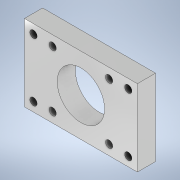
# Autodesk Inventor part: Techo Espaciador Sub. Inferior
Saved by Autodesk Inventor 2020 (Build 240168000, 168)
## iProperties
Created: 2020-05-16
Part Number: Techo Espaciador Sub. Inferior
Material: Aluminum 6061
Document SubType Name: Modeling
Designer: Dante
Density: 2.7 g/cm^3
Appearance: Aluminum - Dark
Mass: 53.2586 g
Surface Area: 78.472 cm^2
Volume: 19.7254 cm^3
Author: Dante
Autodesk Inventor part; units mm, degrees
ref_plane "YZ Plane" through (0, 0, 0) normal (1, 0, 0) x (0, 1, 0)
ref_plane "XZ Plane" through (0, 0, 0) normal (0, 1, 0) x (-1, 0, 0)
ref_plane "XY Plane" through (0, 0, 0) normal (0, 0, 1) x (1, 0, 0)
sketch "Sketch1" plane through (0, 0, 0) normal (0, 0, 1) x (1, 0, 0)
  line L0 (0, 0) -> (0, -42)
  line L1 (0, -42) -> (62, -42)
  line L2 (62, -42) -> (62, 0)
  line L3 (62, 0) -> (0, 0)
  line L4 (11, -42) -> (53, -42)
  line L5 (53, 0) -> (11, 0)
  line L6 (10, -5.9896) -> (10, -30.0104)
  line L7 (31, 0) -> (31, -13)
  circle A0 centre (5, -5) radius 2
  line L8 (0, -21) -> (-21.0238, -21)
  circle A1 centre (31, -21) radius 13
  circle A2 centre (15.5, -5.5) radius 2
  circle A3 centre (15.5, -36.5) radius 2
  circle A4 centre (5, -37) radius 2
  line L9 (52, -5.9896) -> (52, -30.0104)
  circle A5 centre (57, -5) radius 2
  circle A6 centre (46.5, -5.5) radius 2
  circle A7 centre (46.5, -36.5) radius 2
  circle A8 centre (57, -37) radius 2
  dimension "d0" = 42
  dimension "d1" = 62
  dimension "d42" = 10
  dimension "d43" = 4
  dimension "d44" = 5
  dimension "d45" = 5
  dimension "d46" = 26
  dimension "d47" = 4
  dimension "d50" = 4
  dimension "d51" = 5.5
  dimension "d52" = 5.5
  dimension "d53" = 5.5
  dimension "d54" = 31
  constraints: 20 end point, 9 centre point, 7 symmetric about line, 4 perpendicular, 2 vertical, 1 horizontal, 1 midpoint, 1 parallel, 1 point on line, 5 other
  measures "d0" distance of L0.start L0.end
  measures "d1" distance of L0.end L1.end
  measures "d42" distance between parallel lines of L0 L6
  measures "d43" diameter of A0
  measures "d44" distance from line of A0.centre L6
  measures "d45" distance from line of L3 A0.centre
  measures "d46" diameter of A1
  measures "d47" diameter of A2
  measures "d50" diameter of A3
  measures "d51" distance from line of L1 A3.centre
  measures "d52" distance from line of L6 A3.centre
  measures "d53" distance from line of L6 A2.centre
  measures "d54" distance of A3.centre A2.centre
extrude "Extrusion4" add sketch "Sketch1" along normal blind 10
thread "Rosca1" size "M4x0.7" class "6H" standard "ISO Metric profile" length 430
thread "Rosca2" size "M4x0.7" class "6H" standard "ISO Metric profile" length 430
thread "Rosca3" size "M4x0.7" class "6H" standard "ISO Metric profile" length 430
thread "Rosca4" size "M4x0.7" class "6H" standard "ISO Metric profile" length 430
body "Solid3"
